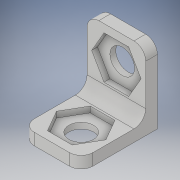
# Autodesk Inventor part: 24 bevestigings hoekjes 2 kanten
Saved by Autodesk Inventor 2019 (Build 230136000, 136)
## iProperties
Created: 2021-05-25
Part Number: 24 bevestigings hoekjes 2 kanten
Material: Generic
Document SubType Name: Modeling
Designer: semboonen
Density: 1 g/cm^3
Appearance: Default
Author: semboonen
Autodesk Inventor part; units mm, degrees
ref_plane "YZ Plane" through (0, 0, 0) normal (1, 0, 0) x (0, 1, 0)
ref_plane "XZ Plane" through (0, 0, 0) normal (0, 1, 0) x (-1, 0, 0)
ref_plane "XY Plane" through (0, 0, 0) normal (0, 0, 1) x (1, 0, 0)
sketch "Sketch1" plane through (0, 0, 0) normal (0, 0, 1) x (1, 0, 0)
  line L0 (-5, -6.5) -> (5, -6.5)
  line L1 (5, -6.5) -> (5, 6.5)
  line L2 (5, 6.5) -> (-5, 6.5)
  line L3 (-5, 6.5) -> (-5, -6.5)
  line L4 (-5, -6.5) -> (5, 6.5) construction
  line L5 (5, -6.5) -> (-5, 6.5) construction
  circle A0 centre (0, 1.5) radius 2.1
  point P0 (0, 0)
  dimension "d0" = 10
  dimension "d1" = 13
  dimension "d2" = 4.2
  dimension "d3" = 5
  dimension "d4" = 5
  constraints: 12 end point, 2 midpoint, 2 parallel, 1 centre point, 1 horizontal, 1 perpendicular
  measures "d0" distance of L2.end L1.end
  measures "d1" distance of L1.end L0.end
  measures "d2" diameter of A0
  measures "d3" distance from line of A0.centre L2
  measures "d4" distance from line of L3 A0.centre
extrude "Extrusion1" add sketch "Sketch1" along normal blind 2
sketch "Sketch2" plane through (-5, -6.5, 0) normal (0, -1, 0) x (1, 0, 0)
  line L0 (0, 0) -> (10, 0)
  line L1 (10, 0) -> (10, 13)
  line L2 (10, 13) -> (0, 13)
  line L3 (0, 13) -> (0, 0)
  circle A0 centre (5, 8) radius 2.1
  point P0 (5, 0)
  dimension "d7" = 10
  dimension "d8" = 13
  dimension "d9" = 5
  dimension "d10" = 13
  dimension "d11" = 4.2
  dimension "d12" = 5
  dimension "d13" = 5
  constraints: 8 end point, 2 parallel, 1 centre point, 1 horizontal, 1 perpendicular
  measures "d7" distance of L2.end L1.end
  measures "d8" distance of L1.end L0.end
  measures "d9" distance from line of point (5, 0) L1
  measures "d10" distance from line of point (5, 0) L2
  measures "d11" diameter of A0
  measures "d12" distance from line of L2 A0.centre
  measures "d13" distance from line of A0.centre L1
extrude "Extrusion2" add sketch "Sketch2" against normal blind 2
sketch "Sketch3" plane through (-5, -4.5, 0) normal (0, 1, 0) x (1, 0, 0)
  circle A0 centre (5, -8) radius 2.1 projected
  line L0 (9.2147, -8) -> (7.1073, -11.65)
  line L1 (7.1073, -11.65) -> (2.8927, -11.65)
  line L2 (2.8927, -11.65) -> (0.7853, -8)
  line L3 (0.7853, -8) -> (2.8927, -4.35)
  line L4 (2.8927, -4.35) -> (7.1073, -4.35)
  line L5 (7.1073, -4.35) -> (9.2147, -8)
  point P0 (5, 0)
  dimension "d16" = 7.3
  constraints: 12 end point, 1 coincident, 1 horizontal, 13 other
  measures "d16" distance between parallel lines of L1 L4
extrude "Extrusion3" cut sketch "Sketch3" against normal blind 1
sketch "Sketch4" plane through (0, 0, 2) normal (0, 0, 1) x (1, 0, 0)
  circle A0 centre (0, 1.5) radius 2.1 projected
  line L0 (4.2147, 1.5) -> (2.1073, -2.15)
  line L1 (2.1073, -2.15) -> (-2.1073, -2.15)
  line L2 (-2.1073, -2.15) -> (-4.2147, 1.5)
  line L3 (-4.2147, 1.5) -> (-2.1073, 5.15)
  line L4 (-2.1073, 5.15) -> (2.1073, 5.15)
  line L5 (2.1073, 5.15) -> (4.2147, 1.5)
  point P0 (0, 0)
  dimension "d19" = 7.3
  constraints: 12 end point, 1 coincident, 1 horizontal, 13 other
  measures "d19" distance between parallel lines of L1 L4
extrude "Extrusion4" cut sketch "Sketch4" against normal blind 1
fillet "Fillet1" radius 2 4 edges at (-5, 6.5, 1) (5, 6.5, 1) (5, -5.5, 13) (-5, -5.5, 13)
fillet "Fillet2" radius 2 1 edges at (0, -4.5, 2)
body "Solid1"
